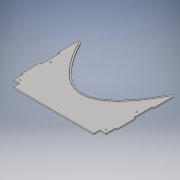
# Autodesk Inventor part: vrRig_v01r1_bottom
Saved by Autodesk Inventor 2016 (Build 200138000, 138)
## iProperties
Created: 2018-01-12
Part Number: vrRig_v01r1_bottom
Material: Generic
Document SubType Name: Modeling
Designer: harveylab
Density: 1 g/cm^3
Appearance: Default
Author: harveylab
Autodesk Inventor part; units mm, degrees
ref_plane "YZ Plane" through (0, 0, 0) normal (1, 0, 0) x (0, 1, 0)
ref_plane "XZ Plane" through (0, 0, 0) normal (0, 1, 0) x (-1, 0, 0)
ref_plane "XY Plane" through (0, 0, 0) normal (0, 0, 1) x (1, 0, 0)
sketch "Sketch2" plane through (0, 0, 0) normal (0, 1, 0) x (-1, 0, 0)
  circle A0 centre (19.05, 261.145) radius 3.302 construction
  circle A1 centre (19.05, 134.145) radius 3.302 construction
  arc A2 (0, 6.35) -> (11.945, 3.3468) centre (6.35, 6.35) ccw
  line L0 (11.945, 3.3468) -> (14.4765, 8.063)
  line L1 (14.4765, 8.063) -> (16.9988, 12.699)
  line L2 (16.9988, 12.699) -> (19.5209, 17.2691)
  line L3 (19.5209, 17.2691) -> (22.0424, 21.7776)
  line L4 (22.0424, 21.7776) -> (24.5631, 26.2191)
  line L5 (24.5631, 26.2191) -> (27.0836, 30.5984)
  line L6 (27.0836, 30.5984) -> (29.6033, 34.9133)
  line L7 (29.6033, 34.9133) -> (32.1222, 39.1641)
  line L8 (32.1222, 39.1641) -> (34.6405, 43.3507)
  line L9 (34.6405, 43.3507) -> (37.158, 47.4731)
  line L10 (37.158, 47.4731) -> (39.6748, 51.5314)
  line L11 (39.6748, 51.5314) -> (42.1907, 55.5255)
  line L12 (42.1907, 55.5255) -> (44.7059, 59.4554)
  line L13 (44.7059, 59.4554) -> (47.2201, 63.3211)
  line L14 (47.2201, 63.3211) -> (49.7335, 67.1225)
  line L15 (49.7335, 67.1225) -> (52.2459, 70.8598)
  line L16 (52.2459, 70.8598) -> (54.7574, 74.5328)
  line L17 (54.7574, 74.5328) -> (57.2678, 78.1415)
  line L18 (57.2678, 78.1415) -> (59.7775, 81.6864)
  line L19 (59.7775, 81.6864) -> (62.2854, 85.1675)
  line L20 (62.2854, 85.1675) -> (64.7926, 88.5822)
  line L21 (64.7926, 88.5822) -> (67.2985, 91.9351)
  line L22 (67.2985, 91.9351) -> (69.8031, 95.2212)
  line L23 (69.8031, 95.2212) -> (72.3065, 98.4455)
  line L24 (72.3065, 98.4455) -> (74.8077, 101.602)
  line L25 (74.8077, 101.602) -> (77.3091, 104.6962)
  line L26 (77.3091, 104.6962) -> (79.809, 107.7286)
  line L27 (79.809, 107.7286) -> (82.3057, 110.6947)
  line L28 (82.3057, 110.6947) -> (84.8017, 113.5951)
  line L29 (84.8017, 113.5951) -> (87.296, 116.4336)
  line L30 (87.296, 116.4336) -> (89.7886, 119.2053)
  line L31 (89.7886, 119.2053) -> (92.2793, 121.9153)
  line L32 (92.2793, 121.9153) -> (94.7682, 124.5585)
  line L33 (94.7682, 124.5585) -> (97.2551, 127.1399)
  line L34 (97.2551, 127.1399) -> (99.7389, 129.6535)
  line L35 (99.7389, 129.6535) -> (102.2229, 132.1051)
  line L36 (102.2229, 132.1051) -> (104.7035, 134.494)
  line L37 (104.7035, 134.494) -> (107.1818, 136.8162)
  line L38 (107.1818, 136.8162) -> (109.6591, 139.078)
  line L39 (109.6591, 139.078) -> (112.1314, 141.2733)
  line L40 (112.1314, 141.2733) -> (114.6011, 143.4022)
  line L41 (114.6011, 143.4022) -> (117.0709, 145.4695)
  line L42 (117.0709, 145.4695) -> (119.5382, 147.4754)
  line L43 (119.5382, 147.4754) -> (121.9997, 149.415)
  line L44 (121.9997, 149.415) -> (124.4599, 151.2897)
  line L45 (124.4599, 151.2897) -> (126.9171, 153.1031)
  line L46 (126.9171, 153.1031) -> (129.3714, 154.8506)
  line L47 (129.3714, 154.8506) -> (131.8225, 156.5369)
  line L48 (131.8225, 156.5369) -> (134.2706, 158.1575)
  line L49 (134.2706, 158.1575) -> (136.7154, 159.7173)
  line L50 (136.7154, 159.7173) -> (139.1569, 161.2116)
  line L51 (139.1569, 161.2116) -> (141.5952, 162.6452)
  line L52 (141.5952, 162.6452) -> (144.0301, 164.0137)
  line L53 (144.0301, 164.0137) -> (146.4616, 165.3218)
  line L54 (146.4616, 165.3218) -> (148.8897, 166.565)
  line L55 (148.8897, 166.565) -> (151.3144, 167.7483)
  line L56 (151.3144, 167.7483) -> (153.7333, 168.8658)
  line L57 (153.7333, 168.8658) -> (156.1536, 169.9235)
  line L58 (156.1536, 169.9235) -> (158.5707, 170.9218)
  line L59 (158.5707, 170.9218) -> (160.9795, 171.8563)
  line L60 (160.9795, 171.8563) -> (163.3876, 172.7281)
  line L61 (163.3876, 172.7281) -> (165.7926, 173.541)
  line L62 (165.7926, 173.541) -> (168.1918, 174.2895)
  line L63 (168.1918, 174.2895) -> (170.5936, 174.9789)
  line L64 (170.5936, 174.9789) -> (172.99, 175.6091)
  line L65 (172.99, 175.6091) -> (175.3838, 176.1764)
  line L66 (175.3838, 176.1764) -> (177.7753, 176.6858)
  line L67 (177.7753, 176.6858) -> (180.1646, 177.1326)
  line L68 (180.1646, 177.1326) -> (182.555, 177.5222)
  line L69 (182.555, 177.5222) -> (184.9376, 177.851)
  line L70 (184.9376, 177.851) -> (187.3187, 178.1177)
  line L71 (187.3187, 178.1177) -> (189.7049, 178.3253)
  line L72 (189.7049, 178.3253) -> (192.0903, 178.4756)
  line L73 (192.0903, 178.4756) -> (194.4687, 178.566)
  line L74 (194.4687, 178.566) -> (196.9262, 178.5955)
  line L75 (196.9262, 178.5955) -> (199.2313, 178.566)
  line L76 (199.2313, 178.566) -> (201.6098, 178.4756)
  line L77 (201.6098, 178.4756) -> (203.9951, 178.3253)
  line L78 (203.9951, 178.3253) -> (206.3813, 178.1177)
  line L79 (206.3813, 178.1177) -> (208.7625, 177.851)
  line L80 (208.7625, 177.851) -> (211.145, 177.5222)
  line L81 (211.145, 177.5222) -> (213.5355, 177.1326)
  line L82 (213.5355, 177.1326) -> (215.9248, 176.6858)
  line L83 (215.9248, 176.6858) -> (218.3162, 176.1764)
  line L84 (218.3162, 176.1764) -> (220.71, 175.6091)
  line L85 (220.71, 175.6091) -> (223.1064, 174.9789)
  line L86 (223.1064, 174.9789) -> (225.5083, 174.2895)
  line L87 (225.5083, 174.2895) -> (227.9074, 173.541)
  line L88 (227.9074, 173.541) -> (230.3124, 172.7281)
  line L89 (230.3124, 172.7281) -> (232.7205, 171.8563)
  line L90 (232.7205, 171.8563) -> (235.1293, 170.9218)
  line L91 (235.1293, 170.9218) -> (237.5464, 169.9235)
  line L92 (237.5464, 169.9235) -> (239.9667, 168.8658)
  line L93 (239.9667, 168.8658) -> (242.3857, 167.7483)
  line L94 (242.3857, 167.7483) -> (244.8103, 166.565)
  line L95 (244.8103, 166.565) -> (247.2385, 165.3218)
  line L96 (247.2385, 165.3218) -> (249.67, 164.0137)
  line L97 (249.67, 164.0137) -> (252.1049, 162.6452)
  line L98 (252.1049, 162.6452) -> (254.5431, 161.2116)
  line L99 (254.5431, 161.2116) -> (256.9847, 159.7173)
  line L100 (256.9847, 159.7173) -> (259.4295, 158.1575)
  line L101 (259.4295, 158.1575) -> (261.8775, 156.5369)
  line L102 (261.8775, 156.5369) -> (264.3286, 154.8506)
  line L103 (264.3286, 154.8506) -> (266.7829, 153.1031)
  line L104 (266.7829, 153.1031) -> (269.2401, 151.2897)
  line L105 (269.2401, 151.2897) -> (271.7003, 149.415)
  line L106 (271.7003, 149.415) -> (274.1618, 147.4754)
  line L107 (274.1618, 147.4754) -> (276.6291, 145.4695)
  line L108 (276.6291, 145.4695) -> (279.099, 143.4022)
  line L109 (279.099, 143.4022) -> (281.5686, 141.2733)
  line L110 (281.5686, 141.2733) -> (284.0409, 139.078)
  line L111 (284.0409, 139.078) -> (286.5182, 136.8162)
  line L112 (286.5182, 136.8162) -> (288.9966, 134.494)
  line L113 (288.9966, 134.494) -> (291.4772, 132.1051)
  line L114 (291.4772, 132.1051) -> (293.9611, 129.6535)
  line L115 (293.9611, 129.6535) -> (296.4449, 127.1399)
  line L116 (296.4449, 127.1399) -> (298.9318, 124.5585)
  line L117 (298.9318, 124.5585) -> (301.4207, 121.9153)
  line L118 (301.4207, 121.9153) -> (303.9115, 119.2053)
  line L119 (303.9115, 119.2053) -> (306.404, 116.4336)
  line L120 (306.404, 116.4336) -> (308.8983, 113.5951)
  line L121 (308.8983, 113.5951) -> (311.3943, 110.6947)
  line L122 (311.3943, 110.6947) -> (313.891, 107.7286)
  line L123 (313.891, 107.7286) -> (316.391, 104.6962)
  line L124 (316.391, 104.6962) -> (318.8923, 101.602)
  line L125 (318.8923, 101.602) -> (321.3936, 98.4455)
  line L126 (321.3936, 98.4455) -> (323.8969, 95.2212)
  line L127 (323.8969, 95.2212) -> (326.4016, 91.9351)
  line L128 (326.4016, 91.9351) -> (328.9075, 88.5822)
  line L129 (328.9075, 88.5822) -> (331.4146, 85.1675)
  line L130 (331.4146, 85.1675) -> (333.9225, 81.6864)
  line L131 (333.9225, 81.6864) -> (336.4322, 78.1415)
  line L132 (336.4322, 78.1415) -> (338.9427, 74.5328)
  line L133 (338.9427, 74.5328) -> (341.4541, 70.8598)
  line L134 (341.4541, 70.8598) -> (343.9665, 67.1225)
  line L135 (343.9665, 67.1225) -> (346.4799, 63.3211)
  line L136 (346.4799, 63.3211) -> (348.9942, 59.4554)
  line L137 (348.9942, 59.4554) -> (351.5093, 55.5255)
  line L138 (351.5093, 55.5255) -> (354.0253, 51.5314)
  line L139 (354.0253, 51.5314) -> (356.542, 47.4731)
  line L140 (356.542, 47.4731) -> (359.0595, 43.3507)
  line L141 (359.0595, 43.3507) -> (361.5778, 39.1641)
  line L142 (361.5778, 39.1641) -> (364.0968, 34.9133)
  line L143 (364.0968, 34.9133) -> (366.6164, 30.5984)
  line L144 (366.6164, 30.5984) -> (369.1369, 26.2191)
  line L145 (369.1369, 26.2191) -> (371.6576, 21.7776)
  line L146 (371.6576, 21.7776) -> (374.1791, 17.2691)
  line L147 (374.1791, 17.2691) -> (376.7012, 12.699)
  line L148 (376.7012, 12.699) -> (379.2236, 8.063)
  line L149 (379.2236, 8.063) -> (381.7551, 3.3468)
  arc A3 (381.7551, 3.3468) -> (393.7, 6.35) centre (387.35, 6.35) ccw
  line L150 (393.7, 6.35) -> (393.7, 7.145)
  line L151 (393.7, 7.145) -> (393.7, 83.345)
  line L152 (393.7, 83.345) -> (387.35, 83.345)
  line L153 (387.35, 83.345) -> (387.35, 159.545)
  line L154 (387.35, 159.545) -> (393.7, 159.545)
  line L155 (393.7, 159.545) -> (393.7, 235.745)
  line L156 (393.7, 235.745) -> (387.35, 235.745)
  line L157 (387.35, 235.745) -> (387.35, 273.845)
  line L158 (387.35, 273.845) -> (361.95, 273.845)
  line L159 (361.95, 273.845) -> (361.95, 299.245)
  line L160 (361.95, 299.245) -> (196.85, 299.245)
  line L161 (196.85, 299.245) -> (31.75, 299.245)
  line L162 (31.75, 299.245) -> (31.75, 273.845)
  line L163 (31.75, 273.845) -> (6.35, 273.845)
  line L164 (6.35, 273.845) -> (6.35, 235.745)
  line L165 (6.35, 235.745) -> (0, 235.745)
  line L166 (0, 235.745) -> (0, 159.545)
  line L167 (0, 159.545) -> (6.35, 159.545)
  line L168 (6.35, 159.545) -> (6.35, 83.345)
  line L169 (6.35, 83.345) -> (0, 83.345)
  line L170 (0, 83.345) -> (0, 7.145)
  line L171 (384.1396, 10.7197) -> (386.6786, 5.9896)
  line L172 (386.6786, 5.9896) -> (387.35, 6.35)
  line L173 (387.35, 6.35) -> (384.81, 11.082)
  line L174 (384.81, 11.082) -> (382.27, 15.7505)
  line L175 (382.27, 15.7505) -> (379.73, 20.353)
  line L176 (379.73, 20.353) -> (377.19, 24.8945)
  line L177 (377.19, 24.8945) -> (374.65, 29.37)
  line L178 (374.65, 29.37) -> (372.11, 33.7833)
  line L179 (372.11, 33.7833) -> (369.57, 38.133)
  line L180 (369.57, 38.133) -> (367.03, 42.4193)
  line L181 (367.03, 42.4193) -> (364.49, 46.642)
  line L182 (364.49, 46.642) -> (361.95, 50.8013)
  line L183 (361.95, 50.8013) -> (359.41, 54.897)
  line L184 (359.41, 54.897) -> (356.87, 58.9293)
  line L185 (356.87, 58.9293) -> (354.33, 62.898)
  line L186 (354.33, 62.898) -> (351.79, 66.8033)
  line L187 (351.79, 66.8033) -> (349.25, 70.645)
  line L188 (349.25, 70.645) -> (346.71, 74.4233)
  line L189 (346.71, 74.4233) -> (344.17, 78.138)
  line L190 (344.17, 78.138) -> (341.63, 81.7893)
  line L191 (341.63, 81.7893) -> (339.09, 85.377)
  line L192 (339.09, 85.377) -> (336.55, 88.9025)
  line L193 (336.55, 88.9025) -> (334.01, 92.362)
  line L194 (334.01, 92.362) -> (331.47, 95.7605)
  line L195 (331.47, 95.7605) -> (328.93, 99.093)
  line L196 (328.93, 99.093) -> (326.39, 102.3645)
  line L197 (326.39, 102.3645) -> (323.85, 105.57)
  line L198 (323.85, 105.57) -> (321.31, 108.712)
  line L199 (321.31, 108.712) -> (318.77, 111.793)
  line L200 (318.77, 111.793) -> (316.23, 114.8105)
  line L201 (316.23, 114.8105) -> (313.69, 117.762)
  line L202 (313.69, 117.762) -> (311.15, 120.6525)
  line L203 (311.15, 120.6525) -> (308.61, 123.477)
  line L204 (308.61, 123.477) -> (306.07, 126.2405)
  line L205 (306.07, 126.2405) -> (303.53, 128.938)
  line L206 (303.53, 128.938) -> (300.99, 131.5745)
  line L207 (300.99, 131.5745) -> (298.45, 134.145)
  line L208 (298.45, 134.145) -> (295.91, 136.652)
  line L209 (295.91, 136.652) -> (293.37, 139.098)
  line L210 (293.37, 139.098) -> (290.83, 141.478)
  line L211 (290.83, 141.478) -> (288.29, 143.797)
  line L212 (288.29, 143.797) -> (285.75, 146.0525)
  line L213 (285.75, 146.0525) -> (283.21, 148.242)
  line L214 (283.21, 148.242) -> (280.67, 150.368)
  line L215 (280.67, 150.368) -> (278.13, 152.433)
  line L216 (278.13, 152.433) -> (275.59, 154.4345)
  line L217 (275.59, 154.4345) -> (273.05, 156.37)
  line L218 (273.05, 156.37) -> (270.51, 158.2445)
  line L219 (270.51, 158.2445) -> (267.97, 160.053)
  line L220 (267.97, 160.053) -> (265.43, 161.8005)
  line L221 (265.43, 161.8005) -> (262.89, 163.482)
  line L222 (262.89, 163.482) -> (260.35, 165.1025)
  line L223 (260.35, 165.1025) -> (257.81, 166.657)
  line L224 (257.81, 166.657) -> (255.27, 168.1505)
  line L225 (255.27, 168.1505) -> (252.73, 169.578)
  line L226 (252.73, 169.578) -> (250.19, 170.9445)
  line L227 (250.19, 170.9445) -> (247.65, 172.245)
  line L228 (247.65, 172.245) -> (245.11, 173.4845)
  line L229 (245.11, 173.4845) -> (242.57, 174.658)
  line L230 (242.57, 174.658) -> (240.03, 175.768)
  line L231 (240.03, 175.768) -> (237.49, 176.817)
  line L232 (237.49, 176.817) -> (234.95, 177.8025)
  line L233 (234.95, 177.8025) -> (232.41, 178.722)
  line L234 (232.41, 178.722) -> (229.87, 179.5805)
  line L235 (229.87, 179.5805) -> (227.33, 180.373)
  line L236 (227.33, 180.373) -> (224.79, 181.102)
  line L237 (224.79, 181.102) -> (222.25, 181.77)
  line L238 (222.25, 181.77) -> (219.71, 182.372)
  line L239 (219.71, 182.372) -> (217.17, 182.913)
  line L240 (217.17, 182.913) -> (214.63, 183.388)
  line L241 (214.63, 183.388) -> (212.09, 183.802)
  line L242 (212.09, 183.802) -> (209.55, 184.1525)
  line L243 (209.55, 184.1525) -> (207.01, 184.437)
  line L244 (207.01, 184.437) -> (204.47, 184.658)
  line L245 (204.47, 184.658) -> (201.93, 184.818)
  line L246 (201.93, 184.818) -> (199.39, 184.9145)
  line L247 (199.39, 184.9145) -> (196.85, 184.945)
  line L248 (196.85, 184.945) -> (194.31, 184.9145)
  line L249 (194.31, 184.9145) -> (191.77, 184.818)
  line L250 (191.77, 184.818) -> (189.23, 184.658)
  line L251 (189.23, 184.658) -> (186.69, 184.437)
  line L252 (186.69, 184.437) -> (184.15, 184.1525)
  line L253 (184.15, 184.1525) -> (181.61, 183.802)
  line L254 (181.61, 183.802) -> (179.07, 183.388)
  line L255 (179.07, 183.388) -> (176.53, 182.913)
  line L256 (176.53, 182.913) -> (173.99, 182.372)
  line L257 (173.99, 182.372) -> (171.45, 181.77)
  line L258 (171.45, 181.77) -> (168.91, 181.102)
  line L259 (168.91, 181.102) -> (166.37, 180.373)
  line L260 (166.37, 180.373) -> (163.83, 179.5805)
  line L261 (163.83, 179.5805) -> (161.29, 178.722)
  line L262 (161.29, 178.722) -> (158.75, 177.8025)
  line L263 (158.75, 177.8025) -> (156.21, 176.817)
  line L264 (156.21, 176.817) -> (153.67, 175.768)
  line L265 (153.67, 175.768) -> (151.13, 174.658)
  line L266 (151.13, 174.658) -> (148.59, 173.4845)
  line L267 (148.59, 173.4845) -> (146.05, 172.245)
  line L268 (146.05, 172.245) -> (143.51, 170.9445)
  line L269 (143.51, 170.9445) -> (140.97, 169.578)
  line L270 (140.97, 169.578) -> (138.43, 168.1505)
  line L271 (138.43, 168.1505) -> (135.89, 166.657)
  line L272 (135.89, 166.657) -> (133.35, 165.1025)
  line L273 (133.35, 165.1025) -> (130.81, 163.482)
  line L274 (130.81, 163.482) -> (128.27, 161.8005)
  line L275 (128.27, 161.8005) -> (125.73, 160.053)
  line L276 (125.73, 160.053) -> (123.19, 158.2445)
  line L277 (123.19, 158.2445) -> (120.65, 156.37)
  line L278 (120.65, 156.37) -> (118.11, 154.4345)
  line L279 (118.11, 154.4345) -> (115.57, 152.433)
  line L280 (115.57, 152.433) -> (113.03, 150.368)
  line L281 (113.03, 150.368) -> (110.49, 148.242)
  line L282 (110.49, 148.242) -> (107.95, 146.0525)
  line L283 (107.95, 146.0525) -> (105.41, 143.797)
  line L284 (105.41, 143.797) -> (102.87, 141.478)
  line L285 (102.87, 141.478) -> (100.33, 139.098)
  line L286 (100.33, 139.098) -> (97.79, 136.652)
  line L287 (97.79, 136.652) -> (95.25, 134.145)
  line L288 (95.25, 134.145) -> (92.71, 131.5745)
  line L289 (92.71, 131.5745) -> (90.17, 128.938)
  line L290 (90.17, 128.938) -> (87.63, 126.2405)
  line L291 (87.63, 126.2405) -> (85.09, 123.477)
  line L292 (85.09, 123.477) -> (82.55, 120.6525)
  line L293 (82.55, 120.6525) -> (80.01, 117.762)
  line L294 (80.01, 117.762) -> (77.47, 114.8105)
  line L295 (77.47, 114.8105) -> (74.93, 111.793)
  line L296 (74.93, 111.793) -> (72.39, 108.712)
  line L297 (72.39, 108.712) -> (69.85, 105.57)
  line L298 (69.85, 105.57) -> (67.31, 102.3645)
  line L299 (67.31, 102.3645) -> (64.77, 99.093)
  line L300 (64.77, 99.093) -> (62.23, 95.7605)
  line L301 (62.23, 95.7605) -> (59.69, 92.362)
  line L302 (59.69, 92.362) -> (57.15, 88.9025)
  line L303 (57.15, 88.9025) -> (54.61, 85.377)
  line L304 (54.61, 85.377) -> (52.07, 81.7893)
  line L305 (52.07, 81.7893) -> (49.53, 78.138)
  line L306 (49.53, 78.138) -> (46.99, 74.4233)
  line L307 (46.99, 74.4233) -> (44.45, 70.645)
  line L308 (44.45, 70.645) -> (41.91, 66.8033)
  line L309 (41.91, 66.8033) -> (39.37, 62.898)
  line L310 (39.37, 62.898) -> (36.83, 58.9293)
  line L311 (36.83, 58.9293) -> (34.29, 54.897)
  line L312 (34.29, 54.897) -> (31.75, 50.8013)
  line L313 (31.75, 50.8013) -> (29.21, 46.642)
  line L314 (29.21, 46.642) -> (26.67, 42.4193)
  line L315 (26.67, 42.4193) -> (24.13, 38.133)
  line L316 (24.13, 38.133) -> (21.59, 33.7833)
  line L317 (21.59, 33.7833) -> (19.05, 29.37)
  line L318 (19.05, 29.37) -> (16.51, 24.8945)
  line L319 (16.51, 24.8945) -> (13.97, 20.353)
  line L320 (13.97, 20.353) -> (11.43, 15.7505)
  line L321 (11.43, 15.7505) -> (8.89, 11.082)
  line L322 (8.89, 11.082) -> (6.35, 6.35)
  line L323 (6.35, 6.35) -> (7.0214, 5.9896)
  line L324 (7.0214, 5.9896) -> (9.5604, 10.7197)
  line L325 (9.5604, 10.7197) -> (12.0983, 15.3844)
  line L326 (12.0983, 15.3844) -> (14.6361, 19.9829)
  line L327 (14.6361, 19.9829) -> (17.1739, 24.5205)
  line L328 (17.1739, 24.5205) -> (19.7116, 28.9919)
  line L329 (19.7116, 28.9919) -> (22.2492, 33.4011)
  line L330 (22.2492, 33.4011) -> (24.7868, 37.7467)
  line L331 (24.7868, 37.7467) -> (27.3243, 42.0286)
  line L332 (27.3243, 42.0286) -> (29.8617, 46.2471)
  line L333 (29.8617, 46.2471) -> (32.399, 50.4019)
  line L334 (32.399, 50.4019) -> (34.9362, 54.4931)
  line L335 (34.9362, 54.4931) -> (37.4733, 58.5208)
  line L336 (37.4733, 58.5208) -> (40.0103, 62.4849)
  line L337 (40.0103, 62.4849) -> (42.5472, 66.3854)
  line L338 (42.5472, 66.3854) -> (45.084, 70.2223)
  line L339 (45.084, 70.2223) -> (47.6207, 73.9956)
  line L340 (47.6207, 73.9956) -> (50.1573, 77.7054)
  line L341 (50.1573, 77.7054) -> (52.6937, 81.3515)
  line L342 (52.6937, 81.3515) -> (55.2301, 84.9341)
  line L343 (55.2301, 84.9341) -> (57.7663, 88.4543)
  line L344 (57.7663, 88.4543) -> (60.3023, 91.9084)
  line L345 (60.3023, 91.9084) -> (62.8382, 95.3015)
  line L346 (62.8382, 95.3015) -> (65.374, 98.6284)
  line L347 (65.374, 98.6284) -> (67.9096, 101.8942)
  line L348 (67.9096, 101.8942) -> (70.4449, 105.0939)
  line L349 (70.4449, 105.0939) -> (72.9803, 108.2301)
  line L350 (72.9803, 108.2301) -> (75.5155, 111.3053)
  line L351 (75.5155, 111.3053) -> (78.0503, 114.3166)
  line L352 (78.0503, 114.3166) -> (80.585, 117.262)
  line L353 (80.585, 117.262) -> (83.1195, 120.1463)
  line L354 (83.1195, 120.1463) -> (85.6538, 122.9644)
  line L355 (85.6538, 122.9644) -> (88.1879, 125.7215)
  line L356 (88.1879, 125.7215) -> (90.7218, 128.4125)
  line L357 (90.7218, 128.4125) -> (93.2554, 131.0424)
  line L358 (93.2554, 131.0424) -> (95.7887, 133.606)
  line L359 (95.7887, 133.606) -> (98.322, 136.1064)
  line L360 (98.322, 136.1064) -> (100.8548, 138.5455)
  line L361 (100.8548, 138.5455) -> (103.3874, 140.9186)
  line L362 (103.3874, 140.9186) -> (105.9199, 143.2307)
  line L363 (105.9199, 143.2307) -> (108.4518, 145.479)
  line L364 (108.4518, 145.479) -> (110.9833, 147.6612)
  line L365 (110.9833, 147.6612) -> (113.5149, 149.7802)
  line L366 (113.5149, 149.7802) -> (116.0462, 151.8381)
  line L367 (116.0462, 151.8381) -> (118.5768, 153.8322)
  line L368 (118.5768, 153.8322) -> (121.1072, 155.7604)
  line L369 (121.1072, 155.7604) -> (123.6373, 157.6276)
  line L370 (123.6373, 157.6276) -> (126.167, 159.4287)
  line L371 (126.167, 159.4287) -> (128.6963, 161.1689)
  line L372 (128.6963, 161.1689) -> (131.2253, 162.8431)
  line L373 (131.2253, 162.8431) -> (133.7539, 164.4563)
  line L374 (133.7539, 164.4563) -> (136.282, 166.0036)
  line L375 (136.282, 166.0036) -> (138.8098, 167.4899)
  line L376 (138.8098, 167.4899) -> (141.3372, 168.9103)
  line L377 (141.3372, 168.9103) -> (143.8642, 170.2698)
  line L378 (143.8642, 170.2698) -> (146.3908, 171.5634)
  line L379 (146.3908, 171.5634) -> (148.9169, 172.7962)
  line L380 (148.9169, 172.7962) -> (151.4424, 173.9629)
  line L381 (151.4424, 173.9629) -> (153.968, 175.0667)
  line L382 (153.968, 175.0667) -> (156.4933, 176.1096)
  line L383 (156.4933, 176.1096) -> (159.0175, 177.089)
  line L384 (159.0175, 177.089) -> (161.5417, 178.0027)
  line L385 (161.5417, 178.0027) -> (164.0655, 178.8558)
  line L386 (164.0655, 178.8558) -> (166.5886, 179.643)
  line L387 (166.5886, 179.643) -> (169.112, 180.3672)
  line L388 (169.112, 180.3672) -> (171.6348, 181.0307)
  line L389 (171.6348, 181.0307) -> (174.1573, 181.6285)
  line L390 (174.1573, 181.6285) -> (176.6794, 182.1657)
  line L391 (176.6794, 182.1657) -> (179.2014, 182.6373)
  line L392 (179.2014, 182.6373) -> (181.7234, 183.0484)
  line L393 (181.7234, 183.0484) -> (184.2445, 183.3964)
  line L394 (184.2445, 183.3964) -> (186.7655, 183.6787)
  line L395 (186.7655, 183.6787) -> (189.287, 183.8981)
  line L396 (189.287, 183.8981) -> (191.8084, 184.0569)
  line L397 (191.8084, 184.0569) -> (194.3291, 184.1527)
  line L398 (194.3291, 184.1527) -> (196.8592, 184.1831)
  line L399 (196.8592, 184.1831) -> (199.371, 184.1527)
  line L400 (199.371, 184.1527) -> (201.8916, 184.0569)
  line L401 (201.8916, 184.0569) -> (204.413, 183.8981)
  line L402 (204.413, 183.8981) -> (206.9346, 183.6787)
  line L403 (206.9346, 183.6787) -> (209.4555, 183.3964)
  line L404 (209.4555, 183.3964) -> (211.9766, 183.0484)
  line L405 (211.9766, 183.0484) -> (214.4987, 182.6373)
  line L406 (214.4987, 182.6373) -> (217.0206, 182.1657)
  line L407 (217.0206, 182.1657) -> (219.5428, 181.6285)
  line L408 (219.5428, 181.6285) -> (222.0652, 181.0307)
  line L409 (222.0652, 181.0307) -> (224.588, 180.3672)
  line L410 (224.588, 180.3672) -> (227.1114, 179.643)
  line L411 (227.1114, 179.643) -> (229.6345, 178.8558)
  line L412 (229.6345, 178.8558) -> (232.1583, 178.0027)
  line L413 (232.1583, 178.0027) -> (234.6825, 177.089)
  line L414 (234.6825, 177.089) -> (237.2067, 176.1096)
  line L415 (237.2067, 176.1096) -> (239.732, 175.0667)
  line L416 (239.732, 175.0667) -> (242.2576, 173.9629)
  line L417 (242.2576, 173.9629) -> (244.7831, 172.7962)
  line L418 (244.7831, 172.7962) -> (247.3092, 171.5634)
  line L419 (247.3092, 171.5634) -> (249.8358, 170.2698)
  line L420 (249.8358, 170.2698) -> (252.3628, 168.9103)
  line L421 (252.3628, 168.9103) -> (254.8902, 167.4899)
  line L422 (254.8902, 167.4899) -> (257.418, 166.0036)
  line L423 (257.418, 166.0036) -> (259.9462, 164.4563)
  line L424 (259.9462, 164.4563) -> (262.4747, 162.8431)
  line L425 (262.4747, 162.8431) -> (265.0037, 161.1689)
  line L426 (265.0037, 161.1689) -> (267.533, 159.4287)
  line L427 (267.533, 159.4287) -> (270.0628, 157.6276)
  line L428 (270.0628, 157.6276) -> (272.5928, 155.7604)
  line L429 (272.5928, 155.7604) -> (275.1232, 153.8322)
  line L430 (275.1232, 153.8322) -> (277.6538, 151.8381)
  line L431 (277.6538, 151.8381) -> (280.1851, 149.7802)
  line L432 (280.1851, 149.7802) -> (282.7167, 147.6612)
  line L433 (282.7167, 147.6612) -> (285.2482, 145.479)
  line L434 (285.2482, 145.479) -> (287.7801, 143.2307)
  line L435 (287.7801, 143.2307) -> (290.3126, 140.9186)
  line L436 (290.3126, 140.9186) -> (292.8452, 138.5455)
  line L437 (292.8452, 138.5455) -> (295.3781, 136.1064)
  line L438 (295.3781, 136.1064) -> (297.9113, 133.606)
  line L439 (297.9113, 133.606) -> (300.4446, 131.0424)
  line L440 (300.4446, 131.0424) -> (302.9782, 128.4125)
  line L441 (302.9782, 128.4125) -> (305.5121, 125.7215)
  line L442 (305.5121, 125.7215) -> (308.0462, 122.9644)
  line L443 (308.0462, 122.9644) -> (310.5805, 120.1463)
  line L444 (310.5805, 120.1463) -> (313.115, 117.262)
  line L445 (313.115, 117.262) -> (315.6497, 114.3166)
  line L446 (315.6497, 114.3166) -> (318.1845, 111.3053)
  line L447 (318.1845, 111.3053) -> (320.7197, 108.2301)
  line L448 (320.7197, 108.2301) -> (323.2551, 105.0939)
  line L449 (323.2551, 105.0939) -> (325.7904, 101.8942)
  line L450 (325.7904, 101.8942) -> (328.326, 98.6284)
  line L451 (328.326, 98.6284) -> (330.8618, 95.3015)
  line L452 (330.8618, 95.3015) -> (333.3977, 91.9084)
  line L453 (333.3977, 91.9084) -> (335.9338, 88.4543)
  line L454 (335.9338, 88.4543) -> (338.4699, 84.9341)
  line L455 (338.4699, 84.9341) -> (341.0063, 81.3515)
  line L456 (341.0063, 81.3515) -> (343.5427, 77.7054)
  line L457 (343.5427, 77.7054) -> (346.0793, 73.9956)
  line L458 (346.0793, 73.9956) -> (348.616, 70.2223)
  line L459 (348.616, 70.2223) -> (351.1528, 66.3854)
  line L460 (351.1528, 66.3854) -> (353.6897, 62.4849)
  line L461 (353.6897, 62.4849) -> (356.2267, 58.5208)
  line L462 (356.2267, 58.5208) -> (358.7638, 54.4931)
  line L463 (358.7638, 54.4931) -> (361.3011, 50.4019)
  line L464 (361.3011, 50.4019) -> (363.8384, 46.2471)
  line L465 (363.8384, 46.2471) -> (366.3757, 42.0286)
  line L466 (366.3757, 42.0286) -> (368.9132, 37.7467)
  line L467 (368.9132, 37.7467) -> (371.4508, 33.4011)
  line L468 (371.4508, 33.4011) -> (373.9884, 28.9919)
  line L469 (373.9884, 28.9919) -> (376.5261, 24.5205)
  line L470 (376.5261, 24.5205) -> (379.0639, 19.9829)
  line L471 (379.0639, 19.9829) -> (381.6018, 15.3844)
  line L472 (381.6018, 15.3844) -> (384.1396, 10.7197)
  line L473 (0, 6.35) -> (0, 7.145)
  circle A4 centre (374.65, 134.145) radius 3.302 construction
  circle A5 centre (374.65, 261.145) radius 3.302 construction
  point P0 (0, 0)
  constraints: 948 end point, 6 centre point, 4 point on circle, 4 point on line
sketch "Sketch3" plane through (0, 0, 0) normal (0, 1, 0) x (-1, 0, 0)
  point P0 (0, 0)
  point P1 (374.65, 261.145)
  point P2 (374.65, 134.145)
  point P3 (19.05, 261.145)
  point P4 (19.05, 134.145)
extrude "Extrusion3" add sketch "Sketch2" along normal blind 5.08
hole "Hole1" at (-374.65, 0, 261.145) at (-374.65, 0, 134.145) at (-19.05, 0, 261.145) at (-19.05, 0, 134.145) direction (0, 1, 0) diameter 4.9784 depth 19.05 tip angle 118 thread size "1/4-20 UNC" class "2B" standard "ANSI Unified Screw Threads"
body "Solid3"
